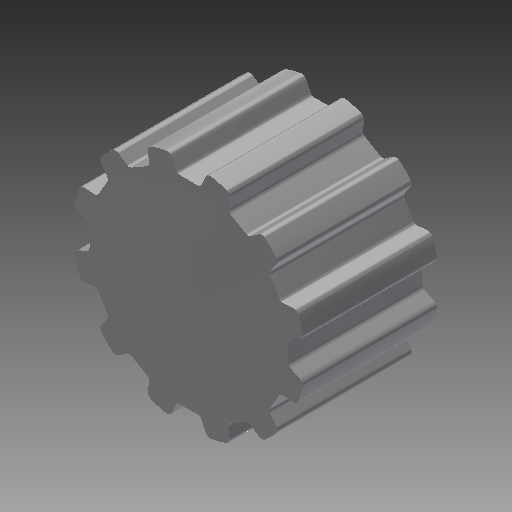
# Autodesk Inventor part: Synchronous Pulley1
Saved by Autodesk Inventor 2017 SP1 (Build 210196100, 196)
## iProperties
Created: 2017-05-14
Part Number: Synchronous Pulley1
Material: Steel
Document SubType Name: Modeling
Designer: Zach
Density: 1 g/cm^3
Appearance: Steel
CustomPartVersion: 1
Author: Zach
Autodesk Inventor part; units mm, degrees
ref_plane "YZ Plane" through (0, 0, 0) normal (1, 0, 0) x (0, 1, 0)
ref_plane "XZ Plane" through (0, 0, 0) normal (0, 1, 0) x (-1, 0, 0)
ref_plane "XY Plane" through (0, 0, 0) normal (0, 0, 1) x (1, 0, 0)
sketch "Pulley Sketch" plane through (0, 0, 0) normal (0, 0, 1) x (1, 0, 0)
  circle A0 centre (0, 0) radius 19.0986 construction
  circle A1 centre (0, 0) radius 18.0986
  circle A2 centre (0, 0) radius 15.4986
  line L0 (-2.9031, 17.8642) -> (-1.8, 15.4986)
  line L1 (-1.8, 15.4986) -> (1.8, 15.4986)
  line L2 (1.8, 15.4986) -> (2.9031, 17.8642)
  line L3 (0, 0) -> (0, 18.0986) construction
  point P0 (0, 15.4986)
  dimension "d0" = 38.1972
  dimension "d1" = 1
  dimension "d2" = 2.6
  dimension "d3" = 50
  dimension "d4" = 3.6
  constraints: 8 end point, 3 coincident, 3 point on circle, 2 centre point, 1 horizontal, 1 midpoint, 1 point on line, 1 vertical, 1 vertical alignment, 3 other
  measures "d0" diameter of A0
  measures "d1" radial gap between concentric circles of A0 A1
  measures "d3" angle of L2 L0
  measures "d4" distance of L0.end L1.end
extrude "Base Body" add sketch "Pulley Sketch" along normal mid plane 21 contours A2 | A1 L0 L1 L2 | L2 L1 L0 A1
extrude "Tooth" cut sketch "Pulley Sketch" along normal through all both and the other way through all contours L2 L1 L0 A1 picked at (0, 17.2145)
fillet "Tooth Fillet" radius 0.6 2 edges at (1.8, 15.4986, 0) (-1.8, 15.4986, 0)
fillet "Tooth Fillet" radius 0.8 4 edges at (-2.9031, 17.8642, 5.25) (-2.9031, 17.8642, -5.25) (2.9031, 17.8642, 5.25) (2.9031, 17.8642, -5.25)
pattern_circular "Teeth" count 12 over 360 about axis through (0, 0, -10) along (0, 0, 1) of "Tooth", "Tooth Fillet"
feature "Left flange" [suppressed]
feature "Right flange" [suppressed]
equation "\"d1\" = da_a"
equation "\"d2\" = da_hg"
equation "\"d3\" = 2 * da_fi"
equation "\"d4\" = da_bw"
equation "\"d5\" = da_bf"
equation "\"d7\" = da_bf"
equation "\"d9\" = da_rb"
equation "\"d10\" = da_rt"
equation "\"da_fi\" = 25deg"
equation "\"da_hg\" = 2.6"
equation "\"da_bw\" = 3.6"
equation "\"da_rb\" = 0.6"
equation "\"da_rt\" = 0.8"
equation "\"da_a\" = 1"
equation "\"da_bf\" = 21"
equation "\"da_wf\" = 1.5"
equation "\"da_hf\" = 1.5"
body "Solid1"
